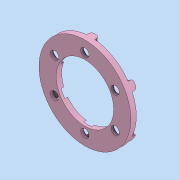
# Autodesk Inventor part: bloque-engrenage
Saved by Autodesk Inventor 2022 (Build 260153000, 153)
## iProperties
Created: 2022-07-29
Part Number: bloque-engrenage
Material: Générique
Document SubType Name: Modeling
Designer: andre
Density: 1 g/cm^3
Appearance: Par défaut(1)
Author: andre
Autodesk Inventor part; units mm, degrees
ref_plane "YZ Plane" through (0, 0, 0) normal (1, 0, 0) x (0, 1, 0)
ref_plane "XZ Plane" through (0, 0, 0) normal (0, 1, 0) x (-1, 0, 0)
ref_plane "XY Plane" through (0, 0, 0) normal (0, 0, 1) x (1, 0, 0)
sketch "Esquisse1" plane through (0, 0, 0) normal (0, 0, 1) x (1, 0, 0)
  circle A0 centre (-22.083648, 0) radius 2.25
  circle A1 centre (-22.083648, 0) radius 1
  arc A2 (-21.041824, -8.290009) -> (-1.041824, -8.290009) centre (-11.041824, 6.375) ccw
  circle A3 centre (-11.041824, 6.375) radius 16.75
  circle A4 centre (-11.041824, -6.375) radius 2.25
  circle A5 centre (0, 0) radius 2.25
  circle A6 centre (0, 12.75) radius 2.25
  circle A7 centre (-11.041824, 19.125) radius 2.25
  circle A8 centre (-22.083648, 12.75) radius 2.25
  circle A9 centre (-11.041824, -6.375) radius 2.25
  circle A10 centre (-11.041824, -6.375) radius 2.25
  circle A11 centre (-11.041824, -6.375) radius 2.25
  circle A12 centre (-11.041824, -6.375) radius 2.75
  circle A13 centre (0, 0) radius 2.75
  circle A14 centre (0, 12.75) radius 2.75
  circle A15 centre (-11.041824, 19.125) radius 2.75
  circle A16 centre (-22.083648, 12.75) radius 2.75
  circle A17 centre (-22.083648, 0) radius 2.75
  dimension "d0" = 1
  dimension "d1" = 0.5
  dimension "d4" = 360
  constraints: 7 centre point, 2 coincident, 13 other
  measures "d0" radial gap between concentric circles of A2 A3
  measures "d1" radial gap between concentric circles of A12 A4
sketch "Esquisse1 outline for Extrusion1" plane through (0, 0, 0) normal (0, 0, 1) x (1, 0, 0)
  circle A0 centre (-11.041824, 6.375) radius 16.75
  circle A1 centre (-11.041824, -6.375) radius 2.75
  circle A2 centre (-22.083648, 0) radius 2.75
  circle A3 centre (0, 0) radius 2.75
  circle A4 centre (-22.083648, 12.75) radius 2.75
  circle A5 centre (0, 12.75) radius 2.75
  circle A6 centre (-11.041824, 19.125) radius 2.75
extrude "Extrusion1" add sketch "Esquisse1 outline for Extrusion1" against normal blind 1
sketch "Esquisse2" plane through (-11.041824, 6.375, -1) normal (0, 0, -1) x (-1, 0, 0)
  circle A0 centre (11.041824, 6.375) radius 2.75
  line L0 (12.271175, 8.834918) -> (13.63779, 9.724874)
  circle A1 centre (0, 0) radius 16.75
  line L1 (13.788658, 6.24308) -> (15.155273, 7.133036)
  circle A2 centre (11.041824, 6.375) radius 2.75
  circle A3 centre (0, 0) radius 16.75
  point P0 (-11.041824, -6.375)
  point P1 (13.788658, 6.24308)
  dimension "d8" = 3
  constraints: 4 end point, 3 point on circle, 2 parallel, 2 other
  measures "d8" distance between parallel lines of L1 L0
sketch "Esquisse2 outline for Extrusion2" plane through (-11.041824, 6.375, -1) normal (0, 0, -1) x (-1, 0, 0)
  line L0 (13.788658, 6.24308) -> (15.155273, 7.133036)
  arc A0 (12.271175, 8.834918) -> (13.788658, 6.24308) centre (11.041824, 6.375) cw
  line L1 (13.63779, 9.724874) -> (12.271175, 8.834918)
  arc A1 (15.155273, 7.133036) -> (13.63779, 9.724874) centre (0, 0) ccw
extrude "Extrusion2" add sketch "Esquisse2 outline for Extrusion2" along normal blind 1.7
fillet "Congé1" radius 1 2 edges at (-23.9963, 15.6549, -2.7) (-25.5138, 13.0631, -2.7)
pattern_circular "Réseau circulaire1" count 6 over 360 about axis through (-11.041824, 6.375, 0) along (0, 0, -1) of "Extrusion2", "Congé1"
sketch "Esquisse3 outline for Extrusion3" plane through (-11.041824, 6.375, 0) normal (0, 0, 1) x (1, 0, 0)
  circle A0 centre (0, 0) radius 16.75
  circle A1 centre (0, -12.75) radius 1.5
  circle A2 centre (-11.041824, -6.375) radius 1.5
  circle A3 centre (11.041824, -6.375) radius 1.5
  circle A4 centre (-11.041824, 6.375) radius 1.5
  circle A5 centre (11.041824, 6.375) radius 1.5
  circle A6 centre (0, 12.75) radius 1.5
extrude "Extrusion3" add sketch "Esquisse3 outline for Extrusion3" along normal blind 1
sketch "Esquisse4" plane through (-11.041824, 6.375, 1) normal (0, 0, 1) x (1, 0, 0)
  circle A0 centre (0, 0) radius 10.5 projected
  point P0 (11.041824, -6.375)
sketch "Esquisse4 outline for Extrusion4" plane through (-11.041824, 6.375, 1) normal (0, 0, 1) x (1, 0, 0)
  circle A0 centre (0, 0) radius 10.5
extrude "Extrusion4" cut sketch "Esquisse4 outline for Extrusion4" against normal up to surface (2 mm away)
